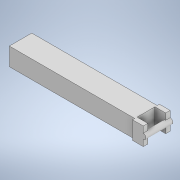
# Autodesk Inventor part: axis_rf
Saved by Autodesk Inventor 2022 (Build 260153000, 153)
## iProperties
Created: 2023-03-23
Part Number: axis_rf
Material: 一般
Document SubType Name: Modeling
Designer: JOU
Density: 1 g/cm^3
Appearance: 預設
Author: JOU
Autodesk Inventor part; units mm, degrees
ref_plane "YZ Plane" through (0, 0, 0) normal (1, 0, 0) x (0, 1, 0)
ref_plane "XZ Plane" through (0, 0, 0) normal (0, 1, 0) x (-1, 0, 0)
ref_plane "XY Plane" through (0, 0, 0) normal (0, 0, 1) x (1, 0, 0)
sketch "草圖1" plane through (0, 0, 0) normal (0, 1, 0) x (-1, 0, 0)
  line L0 (71.0233, 6.25) -> (1.0233, 6.25)
  line L1 (1.0233, 6.25) -> (1.0233, -6.25)
  line L2 (1.0233, -6.25) -> (71.0233, -6.25)
  line L3 (71.0233, -6.25) -> (71.0233, 6.25)
  line L4 (1.0233, 5) -> (-4.9767, 5)
  line L5 (-4.9767, 5) -> (-4.9767, 7.5)
  line L6 (-4.9767, 7.5) -> (1.0233, 7.5)
  line L7 (1.0233, 7.5) -> (1.0233, 5)
  line L8 (1.0233, -5) -> (-4.9767, -5)
  line L9 (-4.9767, -5) -> (-4.9767, -7.5)
  line L10 (-4.9767, -7.5) -> (1.0233, -7.5)
  line L11 (1.0233, -7.5) -> (1.0233, -5)
  point P0 (0, 0)
  point P1 (1.0233, 6.25)
  dimension "d0" = 6
  dimension "d2" = 5
  dimension "d3" = 10
  dimension "d4" = 2.5
  dimension "d5" = 12.5
  dimension "d6" = 6.25
  dimension "d7" = 70
  constraints: 24 end point, 6 parallel, 3 horizontal, 3 perpendicular, 2 collinear, 2 equal length
  measures "d0" distance of L8.start L8.end
  measures "d2" distance from line of point (0, 0) L8
  measures "d3" distance between parallel lines of L8 L4
  measures "d4" distance of L4.end L5.end
  measures "d5" distance of L0.end L1.end
  measures "d6" distance from line of point (0, 0) L2
  measures "d7" distance of L1.end L2.end
extrude "擠出1" add sketch "草圖1" along normal mid plane 10
sketch "草圖2" plane through (-1.0233, 5, 7.5) normal (0, 0, 1) x (1, 0, 0)
  line L0 (6, -10) -> (6, 0) projected
  circle A0 centre (6, -5) radius 1.5
  point P0 (1.0233, -5)
  dimension "d10" = 3
  constraints: 1 centre point, 1 midpoint
  measures "d10" diameter of A0
extrude "擠出2" add sketch "草圖2" against normal up to surface (15 mm away)
equation "\"d6\" = 0.5 * d5"
